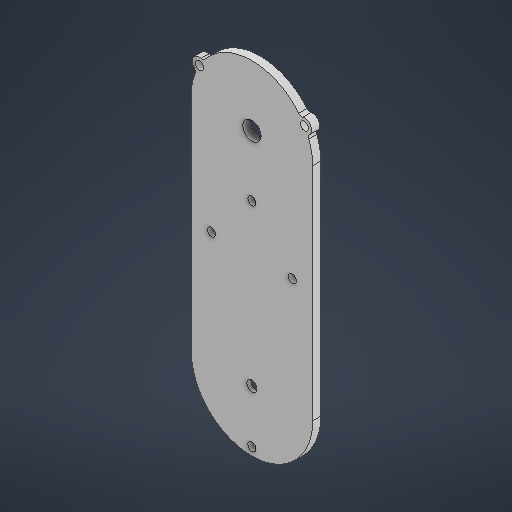
# Autodesk Inventor part: SupNema
Saved by Autodesk Inventor 2025.3 (Build 293356000, 356)
## iProperties
Created: 2025-04-18
Part Number: SupNema
Material: Generic
Document SubType Name: Modeling
Designer: Nelson
Density: 1 g/cm^3
Appearance: Default
Author: Nelson
Autodesk Inventor part; units mm, degrees
ref_plane "YZ Plane" through (0, 0, 0) normal (1, 0, 0) x (0, 1, 0)
ref_plane "XZ Plane" through (0, 0, 0) normal (0, 1, 0) x (-1, 0, 0)
ref_plane "XY Plane" through (0, 0, 0) normal (0, 0, 1) x (1, 0, 0)
sketch "Sketch1" plane through (0, 0, 0) normal (0, 0, 1) x (1, 0, 0)
  circle A0 centre (0, 0) radius 30
  line L0 (0, 0) -> (0, 109.27) construction
  circle A1 centre (0, 109.27) radius 32.5
  line L1 (30, 96.77) -> (30, 0)
  line L2 (-30, 96.77) -> (-30, 0)
  circle A2 centre (0, 0) radius 11
  circle A3 centre (0, 109.27) radius 4.5
  circle A4 centre (0, 109.27) radius 30
  circle A5 centre (0, 79.27) radius 3.5
  line L3 (-30, 96.77) -> (-30, 109.27)
  line L4 (30, 96.77) -> (30, 109.27)
  circle A6 centre (0, 79.27) radius 2
  circle A7 centre (25.9808, 124.27) radius 3.5
  circle A8 centre (25.9808, 124.27) radius 2
  circle A9 centre (-25.9808, 124.27) radius 3.5
  circle A10 centre (-25.9808, 124.27) radius 2
  line L5 (0, 0) -> (0, 55.885) construction
  line L6 (0, 55.885) -> (20, 55.885) construction
  circle A11 centre (20, 55.885) radius 2
  line L7 (0, 55.885) -> (-20, 55.885) construction
  circle A12 centre (-20, 55.885) radius 2
  line L8 (0, -30) -> (0, -26)
  circle A13 centre (0, -26) radius 2
  point P0 (27.551, 121.142)
  point P1 (24.0569, 127.1938)
  point P2 (-24.0569, 127.1938)
  point P3 (-27.551, 121.142)
  dimension "d0" = 60
  dimension "d1" = 109.27
  dimension "d2" = 65
  dimension "d3" = 22
  dimension "d4" = 9
  dimension "d10" = 60
  dimension "Furos" = 7
  dimension "d17" = 4
  dimension "d20" = 360
  dimension "d22" = 55.885
  dimension "d23" = 20
  dimension "d24" = 4
  dimension "d25" = 20
  dimension "d26" = 4
  dimension "d27" = 4
  dimension "d28" = 4
  constraints: 18 end point, 14 centre point, 11 coincident, 8 point on circle, 5 tangent, 3 point on line, 2 vertical, 1 horizontal, 1 perpendicular, 13 other
  measures "d0" diameter of A0
  measures "d1" distance of L0.start L0.end
  measures "d2" diameter of A1
  measures "d3" diameter of A2
  measures "d4" diameter of A3
  measures "d10" diameter of A4
  measures "Furos" diameter of A5
  measures "d17" diameter of A6
  measures "d22" distance of L5.start L5.end
  measures "d23" distance of L5.end L6.end
  measures "d24" diameter of A11
  measures "d25" distance of L5.end L7.end
  measures "d26" diameter of A12
  measures "d27" distance of L8.start L8.end
  measures "d28" diameter of A13
extrude "Extrusion1" add sketch "Sketch1" along normal blind 4 contours A0 | A0 L2 A1 A5 L1 | A1 A5 A4 L4 | L3 A4 A5 A1 | A5 A1 | A1 A5 A4 A6 | A4 A5 A9 A7 | A9 A1 | A1 A9 A4 A10 | A7 A4 A8 A1 | A1 A7 | A7 A4 A8 | A4 A6 A5 | A4 A10 A9
sketch "Sketch2" plane through (0, 0, 4) normal (0, 0, 1) x (1, 0, 0)
  circle A0 centre (0, 0) radius 2.5
  circle A1 centre (0, 0) radius 11
  dimension "d7" = 5
  constraints: 2 centre point, 2 coincident
  measures "d7" diameter of A0
extrude "Extrusion2" add sketch "Sketch2" against normal blind 2
fillet "Fillet1" radius 2 4 edges at (-27.551, 121.142, 2) (-24.0569, 127.1938, 2) (24.0569, 127.1938, 2) (27.551, 121.142, 2)
equation "\"L_Plate\" = d24"
body "Solid1"
